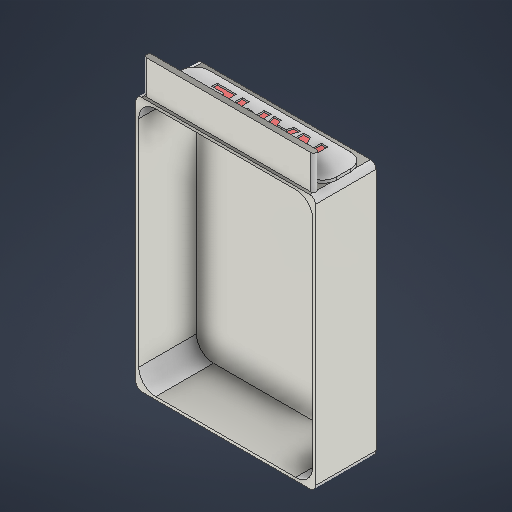
# Autodesk Inventor part: shelf
Saved by Autodesk Inventor 2027 (Build 310192060, 192F)
## iProperties
Created: 2026-06-08
Part Number: shelf
Material: Ogólny
Document SubType Name: Modeling
Designer: User
Density: 1 g/cm^3
Appearance: Domyślna
Author: User
Autodesk Inventor part; units mm, degrees
ref_plane "YZ Plane" through (0, 0, 0) normal (1, 0, 0) x (0, 1, 0)
ref_plane "XZ Plane" through (0, 0, 0) normal (0, 1, 0) x (-1, 0, 0)
ref_plane "XY Plane" through (0, 0, 0) normal (0, 0, 1) x (1, 0, 0)
sketch "Szkic1" plane through (0, 0, 0) normal (0, 1, 0) x (-1, 0, 0)
  line L0 (-31.7, -10.7) -> (31.7, -10.7)
  line L1 (31.7, -10.7) -> (31.7, 10.7)
  line L2 (31.7, 10.7) -> (-31.7, 10.7)
  line L3 (-31.7, 10.7) -> (-31.7, -10.7)
  line L4 (-31.7, -10.7) -> (31.7, 10.7) construction
  line L5 (31.7, -10.7) -> (-31.7, 10.7) construction
  point P0 (0, 0)
  dimension "d0" = 63.4
  dimension "d1" = 21.4
  constraints: 12 end point, 2 midpoint, 2 parallel, 1 horizontal, 1 perpendicular
  measures "d0" distance of L2.end L1.end
  measures "d1" distance of L1.end L0.end
extrude "Wyciągnięcie proste1" add sketch "Szkic1" along normal blind 90
shell "Skorupa1" thickness 1 removed faces 1 at (-10.5667, 30, 10.7)
sketch "Szkic2" plane through (0, 90, 0) normal (0, 1, 0) x (1, 0, 0)
  line L0 (-31.7, -10.7) -> (31.7, -10.7) projected
  line L1 (0, -10.7) -> (0, -8.7)
  line L2 (30, -9.7) -> (-30, -9.7)
  line L3 (-30, -9.7) -> (-30, -7.7)
  line L4 (-30, -7.7) -> (30, -7.7)
  line L5 (30, -7.7) -> (30, -9.7)
  line L6 (30, -9.7) -> (-30, -7.7) construction
  line L7 (-30, -9.7) -> (30, -7.7) construction
  point P0 (0, 0)
  dimension "d5" = 2
  dimension "d6" = 60
  dimension "d7" = 2
  constraints: 14 end point, 3 midpoint, 2 parallel, 1 horizontal, 1 perpendicular, 1 vertical
  measures "d5" distance of L1.start L1.end
  measures "d6" distance of L2.start L2.end
  measures "d7" distance of L2.end L3.end
extrude "Wyciągnięcie proste2" add sketch "Szkic2" along normal blind 12
sketch "Szkic3" plane through (0, 90, 0) normal (0, 1, 0) x (1, 0, 0)
  line L0 (0, 0) -> (0, 1)
  line L1 (30, 8.5) -> (-30, 8.5)
  line L2 (-30, 8.5) -> (-30, -6.5)
  line L3 (-30, -6.5) -> (30, -6.5)
  line L4 (30, -6.5) -> (30, 8.5)
  line L5 (30, 8.5) -> (-30, -6.5) construction
  line L6 (-30, 8.5) -> (30, -6.5) construction
  dimension "d10" = 1
  dimension "d11" = 60
  dimension "d12" = 15
  constraints: 14 end point, 2 midpoint, 2 parallel, 1 horizontal, 1 perpendicular, 1 vertical
  measures "d10" distance of L0.start L0.end
  measures "d11" distance of L3.end L2.end
  measures "d12" distance of L2.end L1.end
extrude "Wyciągnięcie proste3" add sketch "Szkic3" along normal blind 1
sketch "Szkic4" plane through (0, 91, 0) normal (0, 1, 0) x (1, 0, 0)
  line L0 (30, -6.5) -> (-30, -6.5) construction
  line L1 (-30, -6.5) -> (-30, 8.5) construction
  line L2 (-30, 8.5) -> (30, 8.5) construction
  line L3 (30, 8.5) -> (30, -6.5) construction
  line L4 (-30, -6.5) -> (30, -6.5) projected
  line L5 (-30, 8.5) -> (-30, -6.5) projected
  line L6 (30, -6.5) -> (-30, -6.5)
  line L7 (-30, -6.5) -> (-30, 8.5)
  line L8 (-30, 8.5) -> (30, 8.5)
  line L9 (30, 8.5) -> (30, -6.5)
  line L10 (10.778, 6) -> (13.1929, 6)
  line L11 (13.1929, 6) -> (17.0502, -0.9692)
  line L12 (17.0502, -0.9692) -> (17.0502, 6)
  line L13 (17.0502, 6) -> (19.3436, 6)
  line L14 (19.3436, 6) -> (19.3436, -4)
  line L15 (19.3436, -4) -> (16.2642, -4)
  line L16 (16.2642, -4) -> (13.0713, 1.7293)
  line L17 (13.0713, 1.7293) -> (13.0713, -4)
  line L18 (13.0713, -4) -> (10.778, -4)
  line L19 (10.778, -4) -> (10.778, 6)
  line L20 (9.8217, 6) -> (6.4425, -4)
  line L21 (6.4425, -4) -> (3.7034, -4)
  line L22 (3.7034, -4) -> (0.3241, 6)
  line L23 (0.3241, 6) -> (2.9092, 6)
  line L24 (2.9092, 6) -> (3.5332, 3.9579)
  line L25 (3.5332, 3.9579) -> (6.6775, 3.9579)
  line L26 (6.6775, 3.9579) -> (7.3096, 6)
  line L27 (7.3096, 6) -> (9.8217, 6)
  line L28 (4.0843, 2.1426) -> (5.1053, -1.1637)
  line L29 (5.1053, -1.1637) -> (6.1345, 2.1426)
  line L30 (6.1345, 2.1426) -> (4.0843, 2.1426)
  line L31 (-10.8833, 6) -> (-8.3874, 6)
  line L32 (-8.3874, 6) -> (-8.3874, -0.6288)
  line L33 (-8.3874, -0.6288) -> (-6.5721, 3.6499)
  line L34 (-6.5721, 3.6499) -> (-4.8541, 3.6499)
  line L35 (-4.8541, 3.6499) -> (-3.0389, -0.6288)
  line L36 (-3.0389, -0.6288) -> (-3.0389, 6)
  line L37 (-3.0389, 6) -> (-0.6726, 6)
  line L38 (-0.6726, 6) -> (-0.6726, -4)
  line L39 (-0.6726, -4) -> (-3.5656, -4)
  line L40 (-3.5656, -4) -> (-5.7861, 0.9352)
  line L41 (-5.7861, 0.9352) -> (-7.9903, -4)
  line L42 (-7.9903, -4) -> (-10.8833, -4)
  line L43 (-10.8833, -4) -> (-10.8833, 6)
  line L44 (-12.9579, 6) -> (-12.9579, -4)
  line L45 (-12.9579, -4) -> (-19.7164, -4)
  line L46 (-19.7164, -4) -> (-19.7164, -2.0956)
  line L47 (-19.7164, -2.0956) -> (-15.4538, -2.0956)
  line L48 (-15.4538, -2.0956) -> (-15.4538, -0.3371)
  line L49 (-15.4538, -0.3371) -> (-19.3841, -0.3371)
  line L50 (-19.3841, -0.3371) -> (-19.3841, 1.5673)
  line L51 (-19.3841, 1.5673) -> (-15.4538, 1.5673)
  line L52 (-15.4538, 1.5673) -> (-15.4538, 4.0956)
  line L53 (-15.4538, 4.0956) -> (-19.7164, 4.0956)
  line L54 (-19.7164, 4.0956) -> (-19.7164, 6)
  line L55 (-19.7164, 6) -> (-12.9579, 6)
  point P0 (0, 0)
  point P1 (-30, -3.2)
  dimension "d0" = 63.4
  dimension "d1" = 21.4
  constraints: 8 end point, 2 coincident, 2 parallel, 1 horizontal, 1 perpendicular, 2 other
extrude "Wyciągnięcie proste4" cut sketch "Szkic4" against normal blind 0.6 contours L10 L11 L12 L13 L14 L15 L16 L17 L18 L19 | L20 L21 L22 L23 L24 L25 L26 L27 | L31 L32 L33 L34 L35 L36 L37 L38 L39 L40 L41 L42 L43 | L44 L45 L46 L47 L48 L49 L50 L51 L52 L53 L54 L55
fillet "Zaokrąglenie1" radius 5 4 edges at (-30, 90.5, 6.5) (-30, 90.5, -8.5) (30, 90.5, 6.5) (30, 90.5, -8.5)
fillet "Zaokrąglenie2" radius 6 4 edges at (30.7, 1, 0.5) (-30.7, 1, 0.5) (30.7, 89, 0.5) (-30.7, 89, 0.5)
fillet "Zaokrąglenie3" radius 2 4 edges at (31.7, 90, 0) (-31.7, 90, 0) (-31.7, 0, 0) (31.7, 0, 0)
fillet "Zaokrąglenie4" radius 1 4 edges at (-30, 95.9887, 7.7) (-30, 95.9887, 9.7) (30, 95.9887, 7.7) (30, 95.9887, 9.7)
